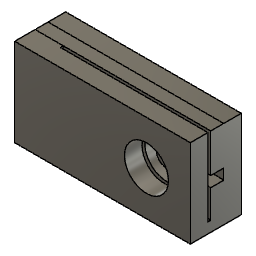
SideWheel_cut v2 (Autodesk Fusion 360 design; units mm, degrees)
Autodesk Fusion 360 part; units mm, degrees
sketch "スケッチ1" plane through (0, 0, 0) normal (0, 0, 1) x (1, 0, 0)
  circle A0 centre (12.5, 12.5) radius 3
  line L0 (18.7913, 13.7566) -> (25, 14)
  line L1 (12.5, 12.5) -> (14, 12.5)
  line L2 (18.7913, 11.2434) -> (25, 11)
  arc A1 (18.5886, 13.9113) -> (18.5886, 11.0887) centre (12.5, 12.5) ccw
  line L3 (25, 0) -> (25, 11)
  line L4 (25, 14) -> (25, 25)
  arc A2 (18.5886, 13.9113) -> (18.7913, 13.7566) centre (18.7834, 13.9564) ccw
  arc A3 (18.7913, 11.2434) -> (18.5886, 11.0887) centre (18.7834, 11.0436) ccw
  line L5 (25, 0) -> (-25, 0)
  line L6 (-25, 0) -> (-25, 25)
  line L7 (-25, 25) -> (25, 25)
  point P0 (18.6237, 13.75)
  point P1 (18.6237, 11.25)
  point P2 (25, 12.5)
  dimension "d3" = 12.5
  dimension "d4" = 6
  dimension "d5" = 2.5
  dimension "d6" = 1.5
  dimension "d7" = 0.2
  dimension "d8" = 0.2
  constraint vertical L3
  constraint concentric A0 A1
  constraint coincident L0.end L3
  constraint coincident A0.centre L1.start
  constraint perpendicular L1 L3
  constraint symmetric L0.end L1 L2.end
  constraint collinear L3 L4
  constraint coincident P2 L3
  constraint coincident P0 L0
  constraint coincident P0 A1
  constraint tangent L0 A2
  constraint tangent A1 A2
  constraint tangent L2 A3
  constraint tangent A1 A3
  constraint perpendicular L3 L5
  constraint perpendicular L5 L6
  measures "d3" diameter of A1
  measures "d4" diameter of A0
  measures "d5" distance of P0 P1
  measures "d6" distance of L0.end P2
  measures "d7" radius of A2
  measures "d8" radius of A3
extrude "押し出し1" add sketch "スケッチ1" along normal blind 4 makes body 1 at (-14.5775, 12.6555, 0) makes body 2 at (15.4963, 12.3505, 2.6667)
sketch "スケッチ2" plane through (0, 0, 0) normal (0, 0, 1) x (1, 0, 0)
  line L0 (-25, 25) -> (25, 25)
  line L1 (25, 25) -> (25, 0)
  line L2 (25, 0) -> (-25, 0)
  line L3 (-25, 0) -> (-25, 25)
  constraint horizontal L0
  constraint vertical L1
  constraint horizontal L2
  constraint vertical L3
extrude "押し出し2" add sketch "スケッチ2" against normal blind 5 separate body makes body 3
sketch "スケッチ3" plane through (0, 0, 0) normal (0, 0, 1) x (1, 0, 0)
  line L0 (-25, 25) -> (-17, 25)
  line L1 (-17, 25) -> (-17, 3)
  line L2 (-17, 0) -> (-25, 0)
  line L3 (-25, 0) -> (-25, 25)
  line L4 (-17, 3) -> (25, 3)
  line L5 (25, 3) -> (25, 0)
  line L6 (25, 0) -> (-17, 0)
  constraint horizontal L0
  constraint vertical L1
  constraint horizontal L2
  constraint vertical L3
  constraint horizontal L4
  constraint vertical L5
  constraint horizontal L6
  constraint coincident L2 L6.end
extrude "押し出し3" add sketch "スケッチ3" along normal blind 1 separate body makes body 4
move_body "移動1" bodies 4 to x (1, 0, 0) y (0, 1, 0) z (0, 0, 1) at (0, 0, 4)
sketch "スケッチ4" plane through (0, 0, 0) normal (0, 0, 1) x (1, 0, 0)
  line L0 (-25, 25) -> (25, 25)
  line L1 (25, 25) -> (25, 0)
  line L2 (25, 0) -> (-25, 0)
  line L3 (-25, 0) -> (-25, 25)
  circle A0 centre (12.5, 12.5) radius 6.25
  dimension "d15" = 12.5
  constraint horizontal L0
  constraint vertical L1
  constraint horizontal L2
  constraint vertical L3
  measures "d15" diameter of A0
extrude "押し出し4" add sketch "スケッチ4" along normal blind 5 separate body makes body 5
move_body "移動2" bodies 5 to x (1, 0, 0) y (0, 1, 0) z (0, 0, 1) at (0, 0, 5)
extrude "押し出し5" cut 1 faces at (-22.3333, 9.3333, 5) along direction (0, 0, -1) blind 0.2 on bodies 4 bodies 4
extrude "押し出し6" cut 2 faces at (-14.5775, 12.6555, 4) (11.4364, 13.3482, 4) along direction (0, 0, -1) blind 0.3 on bodies 1 2 bodies 1 2
move_body "移動3" bodies 4 to x (1, 0, 0) y (0, 1, 0) z (0, 0, 1) at (0, 0, -0.3)
move_body "移動4" bodies 5 to x (1, 0, 0) y (0, 1, 0) z (0, 0, 1) at (0, 0, -0.5)
combine "結合1" operation add target body 3 tool bodies 1
combine "結合2" operation add target body 3 tool bodies 4
combine "結合3" operation add target body 3 tool bodies 5
